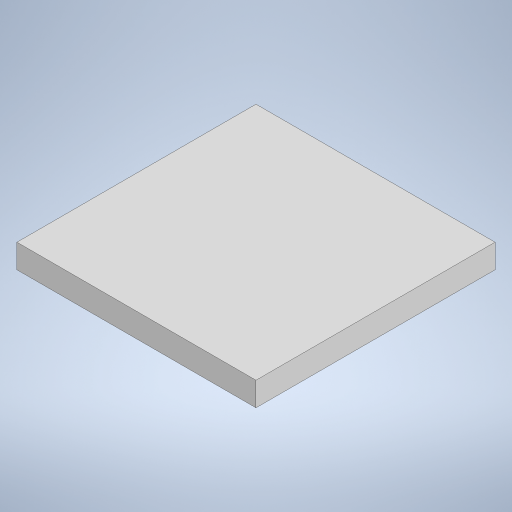
# Autodesk Inventor part: Table
Saved by Autodesk Inventor 2024 (Build 280153000, 153)
## iProperties
Created: 2024-06-18
Part Number: Table
Material: Generic
Document SubType Name: Modeling
Designer: charl
Density: 1 g/cm^3
Appearance: Default
Author: charl
Autodesk Inventor part; units mm, degrees
ref_plane "YZ Plane" through (0, 0, 0) normal (1, 0, 0) x (0, 1, 0)
ref_plane "XZ Plane" through (0, 0, 0) normal (0, 1, 0) x (-1, 0, 0)
ref_plane "XY Plane" through (0, 0, 0) normal (0, 0, 1) x (1, 0, 0)
sketch "Sketch1" plane through (0, 0, 0) normal (0, 1, 0) x (-1, 0, 0)
  line L0 (500, 500) -> (-500, 500)
  line L1 (-500, 500) -> (-500, -500)
  line L2 (-500, -500) -> (500, -500)
  line L3 (500, -500) -> (500, 500)
  point P0 (0, 0)
  dimension "d0" = 1000
  dimension "d1" = 1000
  dimension "d2" = 500
  dimension "d3" = 500
  constraints: 8 end point, 2 parallel, 1 horizontal, 1 perpendicular
  measures "d0" distance of L0.end L1.end
  measures "d1" distance of L1.end L2.end
  measures "d2" distance from line of point (0, 0) L3
  measures "d3" distance from line of point (0, 0) L0
extrude "Extrusion1" add sketch "Sketch1" along normal blind 100
body "Solid1"
